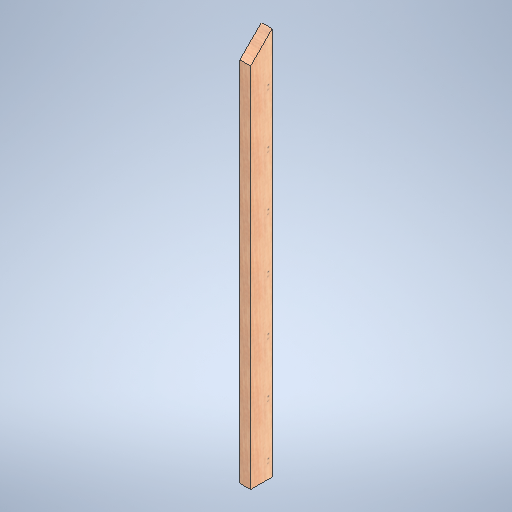
# Autodesk Inventor part: 2x4x72
Saved by Autodesk Inventor 2025 (Build 290162000, 162)
## iProperties
Created: 2024-06-06
Part Number: 2x4x72
Material: Wood (Birch)
Document SubType Name: Modeling
Designer: Cupri
Density: 0.55 g/cm^3
Appearance: Birch - Natural Polished
Author: Cupri
Autodesk Inventor part; units mm, degrees
ref_plane "YZ Plane" through (0, 0, 0) normal (1, 0, 0) x (0, 1, 0)
ref_plane "XZ Plane" through (0, 0, 0) normal (0, 1, 0) x (-1, 0, 0)
ref_plane "XY Plane" through (0, 0, 0) normal (0, 0, 1) x (1, 0, 0)
sketch "Sketch1" plane through (0, 0, 0) normal (0, 1, 0) x (-1, 0, 0)
  line L0 (-25.4, 50.8) -> (25.4, 50.8)
  line L1 (25.4, 50.8) -> (25.4, -50.8)
  line L2 (25.4, -50.8) -> (-25.4, -50.8)
  line L3 (-25.4, -50.8) -> (-25.4, 50.8)
  line L4 (-25.4, 50.8) -> (25.4, -50.8) construction
  line L5 (25.4, 50.8) -> (-25.4, -50.8) construction
  point P0 (0, 0)
  dimension "d0" = 50.8
  dimension "d1" = 101.6
  constraints: 12 end point, 2 midpoint, 2 parallel, 1 horizontal, 1 perpendicular
  measures "d0" distance of L0.start L0.end
  measures "d1" distance of L0.end L1.end
extrude "Extrusion1" add sketch "Sketch1" along normal blind 1828.8
sketch "Sketch2" plane through (25.4, 0, 50.8) normal (1, 0, 0) x (0, 0, -1)
  line L0 (101.6, 1828.8) -> (0, 1828.8) projected
  line L1 (101.6, 1828.8) -> (0, 1727.2)
  line L2 (0, 0) -> (0, 1828.8) projected
  line L3 (0, 1727.2) -> (0, 1828.8)
  line L4 (101.6, 1828.8) -> (0, 1828.8)
  point P0 (50.8, 0)
  dimension "d4" = 45
  constraints: 6 end point, 1 collinear, 1 perpendicular, 1 point on line
  measures "d4" angle of L0 L1
extrude "Extrusion2" cut sketch "Sketch2" against normal blind 50.8
body "Solid1"
